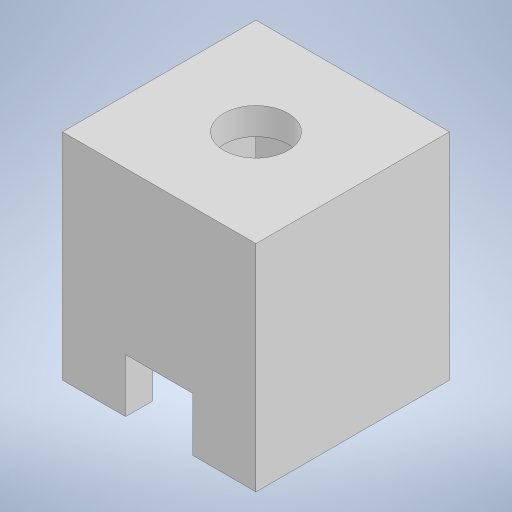
# Autodesk Inventor part: button_holder
Saved by Autodesk Inventor 2023 (Build 270158000, 158)
## iProperties
Created: 2023-10-25
Part Number: button_holder
Material: Generic
Document SubType Name: Modeling
Designer: zskus
Density: 1 g/cm^3
Appearance: Default
Author: zskus
Autodesk Inventor part; units mm, degrees
ref_plane "YZ Plane" through (0, 0, 0) normal (1, 0, 0) x (0, 1, 0)
ref_plane "XZ Plane" through (0, 0, 0) normal (0, 1, 0) x (-1, 0, 0)
ref_plane "XY Plane" through (0, 0, 0) normal (0, 0, 1) x (1, 0, 0)
sketch "Sketch1" plane through (0, 0, 0) normal (0, 1, 0) x (-1, 0, 0)
  line L0 (3.302, 3.302) -> (-3.302, 3.302)
  line L1 (-3.302, 3.302) -> (-3.302, -3.302)
  line L2 (-3.302, -3.302) -> (3.302, -3.302)
  line L3 (3.302, -3.302) -> (3.302, 3.302)
  circle A0 centre (0, 0) radius 1.524
  dimension "d0" = 6.604
  dimension "d1" = 6.604
  dimension "d2" = 3.302
  dimension "d3" = 3.302
  dimension "d6" = 3.048
  constraints: 8 end point, 2 parallel, 1 centre point, 1 coincident, 1 horizontal, 1 perpendicular
  measures "d0" distance of L2.end L0.start
  measures "d1" distance of L0.start L0.end
  measures "d2" distance from line of L0 point (0, 0)
  measures "d3" distance from line of L1 point (0, 0)
  measures "d6" diameter of A0
extrude "Extrusion1" add sketch "Sketch1" along normal blind 1.27
sketch "Sketch2" plane through (0, 1.27, 0) normal (0, 1, 0) x (1, 0, 0)
  line L0 (3.302, -3.302) -> (3.302, 3.302) projected
  line L1 (3.302, 3.302) -> (-3.302, 3.302) projected
  line L2 (-3.302, 3.302) -> (-3.302, -3.302) projected
  line L3 (-3.302, -3.302) -> (3.302, -3.302) projected
  circle A0 centre (0, 0) radius 1.524 projected
  line L4 (-4.572, -4.572) -> (-4.572, 4.572)
  line L5 (-4.572, 4.572) -> (4.572, 4.572)
  line L6 (4.572, 4.572) -> (4.572, -4.572)
  line L7 (4.572, -4.572) -> (-4.572, -4.572)
  dimension "d7" = 1.27
  constraints: 8 end point, 3 other
  measures "d7" distance between parallel lines of L2 L4
extrude "Extrusion2" add sketch "Sketch2" against normal blind 10.16 contours L4 L5 L6 L7
sketch "Sketch3" plane through (-4.572, 1.27, 4.572) normal (0, 0, 1) x (1, 0, 0)
  line L0 (0, 0) -> (9.144, 0) projected
  line L1 (0, 0) -> (0, -10.16) projected
  line L2 (9.144, -10.16) -> (0, -10.16) projected
  line L3 (9.144, 0) -> (9.144, -10.16) projected
  line L4 (0, -10.16) -> (9.144, -10.16) projected
  line L5 (2.9845, -10.16) -> (6.1595, -10.16)
  line L6 (6.1595, -10.16) -> (6.1595, -7.62)
  line L7 (6.1595, -7.62) -> (2.9845, -7.62)
  line L8 (2.9845, -7.62) -> (2.9845, -10.16)
  point P0 (4.572, -1.27)
  point P1 (4.572, -7.62)
  point P2 (2.9845, -10.16)
  dimension "d10" = 3.175
  dimension "d11" = 9.144
  dimension "d12" = 4.572
  dimension "d13" = 2.54
  constraints: 8 end point, 2 parallel, 1 horizontal, 1 midpoint, 1 perpendicular, 1 point on line
  measures "d10" distance of L6.end L7.end
  measures "d11" distance of L0.start L0.end
  measures "d12" distance from line of L3 point (4.572, -7.62)
  measures "d13" distance of L5.end L6.end
extrude "Extrusion3" cut sketch "Sketch3" against normal blind 3.81 contours L8 L7 L6 L2
equation "\"d2\" = 0.5 * d0"
equation "\"d3\" = 0.5 * d1"
equation "\"d12\" = 0.5 * d11"
body "Solid1"
